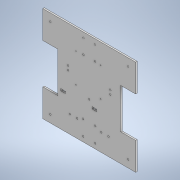
# Autodesk Inventor part: Chassis
Saved by Autodesk Inventor 2020 (Build 240168000, 168)
## iProperties
Created: 2020-02-08
Part Number: Chassis
Material: Generic
Document SubType Name: Modeling
Designer: WIN10
Density: 1 g/cm^3
Appearance: Default
Author: WIN10
Autodesk Inventor part; units mm, degrees
ref_plane "YZ Plane" through (0, 0, 0) normal (1, 0, 0) x (0, 1, 0)
ref_plane "XZ Plane" through (0, 0, 0) normal (0, 1, 0) x (-1, 0, 0)
ref_plane "XY Plane" through (0, 0, 0) normal (0, 0, 1) x (1, 0, 0)
sketch "Sketch1" plane through (0, 0, 0) normal (0, 0, 1) x (1, 0, 0)
  line L0 (-92.5, 40) -> (-92.5, 95)
  line L1 (-92.5, 95) -> (92.5, 95)
  line L2 (92.5, -95) -> (-92.5, -95)
  line L3 (-92.5, -95) -> (-92.5, -40)
  line L4 (-92.5, 95) -> (-62.5, 95)
  line L5 (-62.5, 40) -> (-62.5, -40)
  line L6 (92.5, 95) -> (62.5, 95)
  line L7 (62.5, -15) -> (62.5, 40)
  line L8 (-92.5, 95) -> (-92.5, 40)
  line L9 (-92.5, 40) -> (-62.5, 40)
  line L10 (-92.5, -95) -> (-92.5, -40)
  line L11 (-92.5, -40) -> (-62.5, -40)
  line L12 (62.5, 40) -> (92.5, 40)
  line L13 (62.5, -40) -> (92.5, -40)
  line L14 (92.5, 95) -> (92.5, 40)
  line L15 (92.5, -40) -> (92.5, -95)
  line L16 (-92.5, -95) -> (-77.5, -95)
  line L17 (92.5, -95) -> (77.5, -95)
  line L18 (92.5, 95) -> (77.5, 95)
  line L19 (-92.5, 95) -> (-77.5, 95)
  line L20 (62.5, -40) -> (62.5, -20)
  line L21 (-62.5, -20) -> (-62.5, -40)
  line L22 (-62.5, -20) -> (-62.5, -10)
  line L23 (-62.5, -20) -> (-62.5, -25)
  line L24 (-56.5, -29) -> (-56.5, -25)
  line L25 (-56.5, -25) -> (-47.5, -25)
  line L26 (-47.5, -25) -> (-47.5, -29)
  line L27 (6, -29) -> (6, -25)
  line L28 (15, -25) -> (15, -29)
  line L29 (-47.5, -25) -> (-56.5, -25)
  line L30 (62.5, -20) -> (62.5, -21.75)
  line L31 (62.5, -15) -> (62.5, -21.75)
  line L32 (-56.5, -25) -> (-56.5, -29)
  line L33 (-56.5, -29) -> (-47.5, -29)
  line L34 (6, -29) -> (15, -29)
  line L35 (-62.5, -15) -> (-62.5, -20)
  line L36 (6, -25) -> (15, -25)
  circle A0 centre (-77.5, 80) radius 1.5
  circle A1 centre (77.5, 80) radius 1.5
  circle A2 centre (-77.5, -80) radius 1.5
  circle A3 centre (77.5, -80) radius 1.5
  circle A4 centre (12, -85) radius 1.5
  circle A5 centre (12, -55) radius 1.5
  circle A6 centre (-12, -55) radius 1.5
  circle A7 centre (-12, -85) radius 1.5
  circle A8 centre (-38.5, -60) radius 1.5
  circle A9 centre (-24, -60) radius 1.5
  circle A10 centre (24, -60) radius 1.5
  circle A11 centre (38.5, -60) radius 1.5
  circle A12 centre (0, -15) radius 1.5
  circle A13 centre (42, 14) radius 1.5
  circle A14 centre (42, 22) radius 1.5
  circle A15 centre (-42, 22) radius 1.5
  circle A16 centre (-42, 14) radius 1.5
  circle A17 centre (-11.5, 56) radius 1.5
  circle A18 centre (11.5, 56) radius 1.5
  circle A19 centre (11.5, 85) radius 1.5
  circle A20 centre (-11.5, 85) radius 1.5
  circle A21 centre (-26.5, 54.5) radius 1
  circle A22 centre (22.5, 54.5) radius 1
  circle A23 centre (22.5, -3.5) radius 1
  circle A24 centre (-26.5, -3.5) radius 1
  point P0 (0, 0)
  constraints: 74 end point, 25 centre point, 14 point on line, 10 perpendicular, 3 midpoint, 2 collinear, 2 horizontal
extrude "Extrusion1" add sketch "Sketch1" along normal blind 3
body "Solid1"
